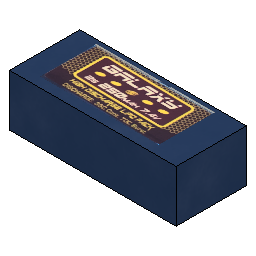
TETRA V10 (Autodesk Fusion 360 archive; units mm, degrees)
design "Galaxy Batteries 2S 250mAh 7.4V LiPoly Pack"
part number: 2026-05-10-15-00-40-955
Autodesk Fusion 360 part; units mm, degrees
sketch "Sketch1" plane through (0, 0, 0) normal (0, 1, 0) x (1, 0, 0)
sketch "Sketch2" plane through (0, 0, 0) normal (0, 1, 0) x (1, 0, 0)
  line L0 (0, 0) -> (45, 0)
  line L1 (45, 0) -> (45, -19)
  line L2 (45, -19) -> (0, -19)
  line L3 (0, -19) -> (0, 0)
  dimension "d1" = 45
  dimension "d2" = 19
  constraint horizontal L0
  constraint vertical L1
  constraint horizontal L2
  constraint vertical L3
  constraint coincident L0.start L3.end
  measures "d1" distance of L0.start L0.end
  measures "d2" distance of L0.start L2.end
extrude "Extrude1" add sketch "Sketch2" along normal blind 14
